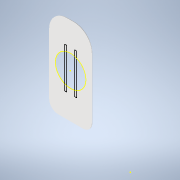
# Autodesk Inventor part: Bodenplatte-Holz
Saved by Autodesk Inventor 2020.3 (Build 243373010, 373A)
## iProperties
Created: 2021-01-31
Part Number: Bodenplatte-Holz
Material: Generisch
Document SubType Name: Modeling
Designer: Stefan
Density: 1 g/cm^3
Appearance: Vorgabe
Author: Stefan
Autodesk Inventor part; units mm, degrees
ref_plane "YZ Plane" through (0, 0, 0) normal (1, 0, 0) x (0, 1, 0)
ref_plane "XZ Plane" through (0, 0, 0) normal (0, 1, 0) x (-1, 0, 0)
ref_plane "XY Plane" through (0, 0, 0) normal (0, 0, 1) x (1, 0, 0)
sketch "Skizze2" plane through (0, 0, 0) normal (0, 0, 1) x (1, 0, 0)
  line L0 (-1807.4619, 517.1639) -> (-1807.4619, 1867.1639)
  line L1 (-1407.4619, 2267.1639) -> (-1257.4619, 2267.1639)
  line L2 (-857.4619, 1867.1639) -> (-857.4619, 517.1639)
  line L3 (-1057.4619, 317.1639) -> (-1607.4619, 317.1639)
  arc A0 (-1407.4619, 2267.1639) -> (-1807.4619, 1867.1639) centre (-1407.4619, 1867.1639) ccw
  arc A1 (-857.4619, 1867.1639) -> (-1257.4619, 2267.1639) centre (-1257.4619, 1867.1639) ccw
  arc A2 (-1807.4619, 517.1639) -> (-1607.4619, 317.1639) centre (-1607.4619, 517.1639) ccw
  arc A3 (-1057.4619, 317.1639) -> (-857.4619, 517.1639) centre (-1057.4619, 517.1639) ccw
  circle A4 centre (-1332.4619, 1292.1639) radius 340
  point P0 (-857.4619, 2267.1639)
  point P1 (-1807.4619, 2267.1639)
  point P2 (-857.4619, 317.1639)
  dimension "d0" = 950
  dimension "d1" = 1950
  dimension "d2" = 400
  dimension "d3" = 200
  dimension "d4" = 680
  dimension "d17" = 475
  dimension "d18" = 975
  constraints: 8 end point, 8 point on circle, 8 tangent, 6 point on line, 5 centre point, 2 equal radius, 2 parallel, 1 coincident, 1 perpendicular, 1 vertical
  measures "d0" distance of point (-1807.462, 2267.164) point (-857.462, 2267.164)
  measures "d1" distance of point (-857.462, 2267.164) point (-857.462, 317.164)
  measures "d2" radius of A0
  measures "d3" radius of A2
  measures "d4" diameter of A4
  measures "d17" distance from line of L0 A4.centre
  measures "d18" distance from line of L1 A4.centre
extrude "Extrusion1" add sketch "Skizze2" along normal blind 10
sketch "Skizze3" plane through (0, 0, 10) normal (0, 0, 1) x (1, 0, 0)
  line L0 (-1202.4619, 1742.1639) -> (-1202.4619, 842.1639)
  line L1 (-1202.4619, 842.1639) -> (-1242.4619, 842.1639)
  line L2 (-1242.4619, 842.1639) -> (-1242.4619, 1742.1639)
  line L3 (-1242.4619, 1742.1639) -> (-1202.4619, 1742.1639)
  line L4 (-1462.4619, 842.1639) -> (-1462.4619, 1742.1639)
  line L5 (-1462.4619, 1742.1639) -> (-1422.4619, 1742.1639)
  line L6 (-1422.4619, 1742.1639) -> (-1422.4619, 842.1639)
  line L7 (-1422.4619, 842.1639) -> (-1462.4619, 842.1639)
  circle A0 centre (-1332.4619, 1292.1639) radius 340 projected
  point P0 (0, 0)
  dimension "d9" = 900
  dimension "d10" = 40
  dimension "d13" = 900
  dimension "d14" = 40
  dimension "d20" = 260
  dimension "d21" = 0
  dimension "d23" = 130
  dimension "d24" = 450
  constraints: 16 end point, 4 parallel, 2 perpendicular, 2 vertical
  measures "d9" distance of L1.end L2.end
  measures "d10" distance of L0.end L1.end
  measures "d13" distance of L5.end L6.end
  measures "d14" distance of L4.end L5.end
  measures "d20" distance between parallel lines of L4 L0
  measures "d21" distance between parallel lines of L1 L7
  measures "d23" distance from line of A0.centre L4
  measures "d24" distance from line of A0.centre L1
